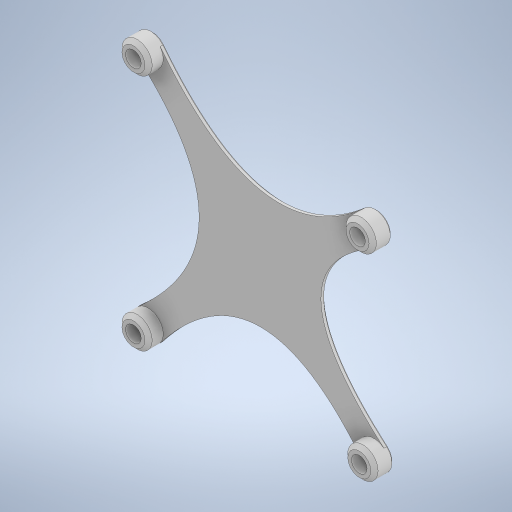
# Autodesk Inventor part: TinyFan_Extrusion_Top
Saved by Autodesk Inventor 2023.1 (Build 271208000, 208)
## iProperties
Created: 2022-09-15
Part Number: TinyFan_Extrusion_Top
Material: Generisch
Document SubType Name: Modeling
Designer: Rama
Density: 1 g/cm^3
Appearance: Vorgabe
Author: Rama
Autodesk Inventor part; units mm, degrees
ref_plane "YZ Plane" through (0, 0, 0) normal (1, 0, 0) x (0, 1, 0)
ref_plane "XZ Plane" through (0, 0, 0) normal (0, 1, 0) x (-1, 0, 0)
ref_plane "XY Plane" through (0, 0, 0) normal (0, 0, 1) x (1, 0, 0)
sketch "Skizze1" plane through (0, 0, 0) normal (0, 0, 1) x (1, 0, 0)
  circle A0 centre (-25.837, 27.4295) radius 1.65 projected
  line L0 (-38.2086, 5.3216) -> (-37.4869, 5.3204) projected
  line L1 (-37.4869, 5.3204) -> (-37.4918, 2.4829) projected
  line L2 (-37.4918, 2.4829) -> (-35.7716, 2.4799) projected
  line L3 (-35.7716, 2.4799) -> (-35.7668, 5.1987) projected
  line L4 (-35.7668, 5.1987) -> (-35.0451, 5.1975) projected
  line L5 (-35.0451, 5.1975) -> (-35.0499, 2.4787) projected
  line L6 (-35.0499, 2.4787) -> (-32.1136, 2.4735) projected
  line L7 (-32.1136, 2.4735) -> (-32.115, 1.6628) projected
  line L8 (-32.115, 1.6628) -> (-38.215, 1.6735) projected
  line L9 (-38.215, 1.6735) -> (-38.2086, 5.3216) projected
  line L10 (-35.0952, -3.6509) -> (-32.1243, -3.6561) projected
  line L11 (-32.1243, -3.6561) -> (-32.1256, -4.4273) projected
  line L12 (-32.1256, -4.4273) -> (-34.7356, -4.4227) projected
  spline S0 degree 2 poles (-34.7356, -4.4227) (-35.052, -4.4222) (-35.5959, -4.4805) (-35.7592, -4.5692) knots 0 0 0 1 2 2 2 projected
  spline S1 degree 2 poles (-35.7592, -4.5692) (-35.9323, -4.6628) (-36.101, -4.9987) (-36.1015, -5.2854) knots 0 0 0 1 2 2 2 projected
  spline S2 degree 2 poles (-36.1015, -5.2854) (-36.102, -5.5721) (-35.7966, -6.1807) (-35.5499, -6.4728) knots 0 0 0 1 2 2 2 projected
  line L13 (-35.5499, -6.4728) -> (-32.1292, -6.4787) projected
  line L14 (-32.1292, -6.4787) -> (-32.1305, -7.2499) projected
  line L15 (-32.1305, -7.2499) -> (-36.708, -7.2419) projected
  line L16 (-36.708, -7.2419) -> (-36.7066, -6.4707) projected
  line L17 (-36.7066, -6.4707) -> (-36.1975, -6.4716) projected
  spline S3 degree 2 poles (-36.1975, -6.4716) (-36.5083, -6.125) (-36.8334, -5.4571) (-36.8327, -5.0815) knots 0 0 0 1 2 2 2 projected
  spline S4 degree 2 poles (-36.8327, -5.0815) (-36.8316, -4.4092) (-35.9405, -3.6495) (-35.0952, -3.6509) knots 0 0 0 1 2 2 2 projected
  line L18 (-36.71, -8.3739) -> (-32.1325, -8.3819) projected
  line L19 (-32.1325, -8.3819) -> (-32.1338, -9.153) projected
  line L20 (-32.1338, -9.153) -> (-36.7113, -9.145) projected
  line L21 (-36.7113, -9.145) -> (-36.71, -8.3739) projected
  line L22 (-32.1384, -11.773) -> (-32.1398, -12.5837) projected
  line L23 (-32.1398, -12.5837) -> (-37.5181, -12.5743) projected
  line L24 (-37.5181, -12.5743) -> (-37.5217, -14.6208) projected
  line L25 (-37.5217, -14.6208) -> (-38.2434, -14.6195) projected
  line L26 (-38.2434, -14.6195) -> (-38.2348, -9.7158) projected
  line L27 (-38.2348, -9.7158) -> (-37.5131, -9.7171) projected
  line L28 (-37.5131, -9.7171) -> (-37.5167, -11.7636) projected
  line L29 (-37.5167, -11.7636) -> (-32.1384, -11.773) projected
  line L30 (-38.2719, -8.3168) -> (-37.4711, -8.3182) projected
  line L31 (-37.4711, -8.3182) -> (-37.4727, -9.1931) projected
  line L32 (-37.4727, -9.1931) -> (-38.2735, -9.1917) projected
  line L33 (-38.2735, -9.1917) -> (-38.2719, -8.3168) projected
  line L34 (-36.695, 0.2274) -> (-36.6936, 1.0282) projected
  line L35 (-36.6936, 1.0282) -> (-30.4347, -1.4445) projected
  line L36 (-30.4347, -1.4445) -> (-30.4362, -2.27) projected
  line L37 (-30.4362, -2.27) -> (-32.3428, -1.4461) projected
  line L38 (-32.3428, -1.4461) -> (-36.7008, -3.0994) projected
  line L39 (-36.7008, -3.0994) -> (-36.6993, -2.269) projected
  line L40 (-36.6993, -2.269) -> (-33.306, -1.0242) projected
  line L41 (-33.306, -1.0242) -> (-36.695, 0.2274) projected
  line L42 (-32.103, 8.529) -> (-32.5874, 8.5299) projected
  spline S5 degree 2 poles (-32.5874, 8.5299) (-32.5184, 8.4358) (-32.2718, 8.119) (-32.1979, 7.9706) knots 0 0 0 1 2 2 2 projected
  spline S6 degree 2 poles (-32.1979, 7.9706) (-32.0895, 7.7677) (-31.9765, 7.3869) (-31.9771, 7.0409) knots 0 0 0 1 2 2 2 projected
  spline S7 degree 2 poles (-31.9771, 7.0409) (-31.9775, 6.7591) (-32.191, 6.2503) (-32.3841, 6.0579) knots 0 0 0 1 2 2 2 projected
  spline S8 degree 2 poles (-32.3841, 6.0579) (-32.5723, 5.8753) (-33.1263, 5.6538) (-33.4328, 5.6544) knots 0 0 0 1 2 2 2 projected
  spline S9 degree 2 poles (-33.4328, 5.6544) (-33.9074, 5.6552) (-34.5789, 6.0568) (-34.771, 6.4921) knots 0 0 0 1 2 2 2 projected
  spline S10 degree 2 poles (-34.771, 6.4921) (-34.9483, 6.878) (-35.0799, 7.9262) (-35.1134, 8.5343) knots 0 0 0 1 2 2 2 projected
  line L43 (-35.1134, 8.5343) -> (-35.2617, 8.5345) projected
  spline S11 degree 2 poles (-35.2617, 8.5345) (-35.5287, 8.535) (-35.8602, 8.3725) (-35.9543, 8.2243) knots 0 0 0 1 2 2 2 projected
  spline S12 degree 2 poles (-35.9543, 8.2243) (-36.0485, 8.0762) (-36.1086, 7.6512) (-36.109, 7.4238) knots 0 0 0 1 2 2 2 projected
  spline S13 degree 2 poles (-36.109, 7.4238) (-36.1094, 7.1569) (-35.9525, 6.4349) (-35.7999, 6.0737) knots 0 0 0 1 2 2 2 projected
  line L44 (-35.7999, 6.0737) -> (-35.8, 6.0292) projected
  line L45 (-35.8, 6.0292) -> (-36.586, 6.0306) projected
  spline S14 degree 2 poles (-36.586, 6.0306) (-36.6449, 6.2433) (-36.7918, 7.0394) (-36.7911, 7.4299) knots 0 0 0 1 2 2 2 projected
  spline S15 degree 2 poles (-36.7911, 7.4299) (-36.7903, 7.9045) (-36.6409, 8.5518) (-36.4476, 8.8085) knots 0 0 0 1 2 2 2 projected
  spline S16 degree 2 poles (-36.4476, 8.8085) (-36.2594, 9.0603) (-35.6608, 9.3064) (-35.2307, 9.3056) knots 0 0 0 1 2 2 2 projected
  line L46 (-35.2307, 9.3056) -> (-32.1016, 9.3002) projected
  line L47 (-32.1016, 9.3002) -> (-32.103, 8.529) projected
  line L48 (-35.0644, 13.9817) -> (-32.0935, 13.9765) projected
  line L49 (-32.0935, 13.9765) -> (-32.0948, 13.2054) projected
  line L50 (-32.0948, 13.2054) -> (-34.7049, 13.2099) projected
  spline S17 degree 2 poles (-34.7049, 13.2099) (-35.0212, 13.2105) (-35.5651, 13.1521) (-35.7284, 13.0634) knots 0 0 0 1 2 2 2 projected
  spline S18 degree 2 poles (-35.7284, 13.0634) (-35.9016, 12.9698) (-36.0702, 12.6339) (-36.0707, 12.3472) knots 0 0 0 1 2 2 2 projected
  spline S19 degree 2 poles (-36.0707, 12.3472) (-36.0712, 12.0605) (-35.7658, 11.452) (-35.5191, 11.1599) knots 0 0 0 1 2 2 2 projected
  line L51 (-35.5191, 11.1599) -> (-32.0984, 11.1539) projected
  line L52 (-32.0984, 11.1539) -> (-32.0998, 10.3828) projected
  line L53 (-32.0998, 10.3828) -> (-36.6772, 10.3907) projected
  line L54 (-36.6772, 10.3907) -> (-36.6759, 11.1619) projected
  line L55 (-36.6759, 11.1619) -> (-36.1667, 11.161) projected
  spline S20 degree 2 poles (-36.1667, 11.161) (-36.4775, 11.5076) (-36.8026, 12.1755) (-36.802, 12.5512) knots 0 0 0 1 2 2 2 projected
  spline S21 degree 2 poles (-36.802, 12.5512) (-36.8008, 13.2235) (-35.9097, 13.9832) (-35.0644, 13.9817) knots 0 0 0 1 2 2 2 projected
  circle A1 centre (-25.837, -24.3815) radius 1.65 projected
  circle A2 centre (22.931, 18.2855) radius 1.65 projected
  circle A3 centre (23.297, -24.3815) radius 1.65 projected
  arc A4 (-37.7973, 28.9208) -> (-39.6082, 27.5864) centre (-37.7217, 26.9222) ccw projected
  arc A5 (-39.6082, 27.5864) -> (-39.8919, 25.917) centre (-34.8919, 25.926) ccw projected
  line L56 (-39.8919, 25.917) -> (-39.8874, 23.4424) projected
  line L57 (-39.8874, 23.4424) -> (-39.478, 23.4424) projected
  arc A6 (-39.478, 21.4424) -> (-39.478, 23.4424) centre (-34.8856, 22.4424) ccw projected
  line L58 (-39.478, 21.4424) -> (-39.8838, 21.4424) projected
  line L59 (-39.8838, 21.4424) -> (-39.8061, -21.5576) projected
  line L60 (-39.8061, -21.5576) -> (-39.3966, -21.5576) projected
  arc A7 (-39.3966, -23.5576) -> (-39.3966, -21.5576) centre (-34.8043, -22.5576) ccw projected
  line L61 (-39.3966, -23.5576) -> (-39.8025, -23.5576) projected
  line L62 (-39.8025, -23.5576) -> (-39.798, -26.0503) projected
  arc A8 (-39.798, -26.0503) -> (-39.5082, -27.7186) centre (-34.798, -26.0413) ccw projected
  arc A9 (-39.5082, -27.7186) -> (-37.6925, -29.0465) centre (-37.6241, -27.0477) ccw projected
  line L63 (-37.6925, -29.0465) -> (-31.8925, -29.036) projected
  spline S22 degree 2 poles (-31.8925, -29.036) (-30.8606, -29.0341) (-25.3454, -28.3512) knots -2 -2 -2 -1 -1 -1 projected
  arc A10 (-25.3454, -28.3512) -> (-22.6346, -26.7782) centre (-25.837, -24.3815) ccw projected
  spline S23 degree 2 poles (-22.6346, -26.7782) (-1.453, 1.524) (20.1144, -26.8045) knots -2 -2 -2 -1 -1 -1 projected
  arc A11 (20.1144, -26.8045) -> (25.8626, -21.3127) centre (23.297, -24.3815) ccw projected
  arc A12 (24.7305, 14.7131) -> (20.2403, 21.2453) centre (22.931, 18.2855) ccw projected
  spline S24 degree 2 poles (20.2403, 21.2453) (-1.453, 1.524) (-22.6346, 29.8262) knots -2 -2 -2 -1 -1 -1 projected
  arc A13 (-22.6346, 29.8262) -> (-27.9876, 30.8022) centre (-25.837, 27.4295) ccw projected
  spline S25 degree 2 poles (-27.9876, 30.8022) (-30.9185, 28.9332) (-31.9973, 28.9313) knots -2 -2 -2 -1 -1 -1 projected
  line L64 (-31.9973, 28.9313) -> (-37.7973, 28.9208) projected
  circle A14 centre (-25.837, 27.4295) radius 1.7
  circle A15 centre (-25.837, -24.3815) radius 1.7
  circle A16 centre (23.297, -24.3815) radius 1.7
  circle A17 centre (22.931, 18.2855) radius 1.7
  circle A18 centre (-25.837, 27.4295) radius 3.3
  circle A19 centre (22.931, 18.2855) radius 3.3
  circle A20 centre (23.297, -24.3815) radius 3.3
  circle A21 centre (-25.837, -24.3815) radius 3.3
  line L65 (-28.0198, -21.9065) -> (-1.453, 1.524) construction
  line L66 (-1.453, 1.524) -> (-28.0198, 24.9545) construction
  spline S26 degree 2 poles (-28.0198, -21.9065) (-1.453, 1.524) (-28.0198, 24.9545) knots 1 1 1 2 2 2
  line L67 (-23.2346, 29.4587) -> (-1.453, 1.524) construction
  line L68 (-1.453, 1.524) -> (20.77, 20.7795) construction
  spline S27 degree 2 poles (-23.2346, 29.4587) (-1.453, 1.524) (20.77, 20.7795) knots 1 1 1 2 2 2
  line L69 (-23.2346, -26.4107) -> (-1.453, 1.524) construction
  line L70 (-1.453, 1.524) -> (20.7111, -26.4317) construction
  spline S28 degree 2 poles (-23.2346, -26.4107) (-1.453, 1.524) (20.7111, -26.4317) knots 1 1 1 2 2 2
  line L71 (25.4629, -21.8918) -> (-1.453, 1.524) construction
  line L72 (-1.453, 1.524) -> (24.4854, 15.3745) construction
  spline S29 degree 2 poles (25.4629, -21.8918) (-1.453, 1.524) (24.4854, 15.3745) knots 1 1 1 2 2 2
  spline S30 degree 2 poles (25.8626, -21.3127) (21.9132, -18.0109) (19.0822, -14.9107) knots -2 -2 -2 -1.855416 -1.855416 -1.855416 projected
  spline S31 degree 2 poles (17.22, 9.815) (18.4126, 10.8679) (19.8732, 11.8725) knots 1.825455 1.825455 1.825455 1.896249 1.896249 1.896249 projected
  spline S32 degree 2 poles (17.22, -12.7436) (6.6116, 0.4487) (17.22, 9.815) knots -1.804293 -1.804293 -1.804293 -1.174545 -1.174545 -1.174545 projected
  spline S33 degree 2 poles (19.8732, 11.8725) (22.0139, 13.3447) (24.7305, 14.7131) knots -1.103751 -1.103751 -1.103751 -1 -1 -1 projected
  spline S34 degree 2 poles (19.0822, -14.9107) (18.0812, -13.8146) (17.22, -12.7436) knots 1.144584 1.144584 1.144584 1.195707 1.195707 1.195707 projected
  point P0 (0, 0)
  point P1 (24.4854, 15.3745)
  point P2 (20.77, 20.7795)
  dimension "d5" = 6.6
  dimension "d0" = 3.4
  dimension "d1" = 3.4
  dimension "d2" = 3.4
  dimension "d3" = 3.4
  dimension "d4" = 1.6
  dimension "d6" = 6.6
  dimension "d7" = 6.6
  dimension "d8" = 6.6
  dimension "d9" = 51.811
  dimension "d10" = 25.9055
  dimension "d11" = 48.768
  dimension "d12" = 24.384
  constraints: 11 coincident, 7 centre point, 21 other
  measures "d0" diameter of A14
  measures "d1" diameter of A15
  measures "d2" diameter of A16
  measures "d3" diameter of A17
  measures "d6" diameter of A19
  measures "d7" diameter of A20
  measures "d8" diameter of A21
  measures "d9" distance of A1.centre A0.centre
  measures "d10" vertical distance of L71.end A1.centre
  measures "d11" horizontal distance of A2.centre A0.centre
  measures "d12" horizontal distance of L67.end A0.centre
extrude "Extrusion1" add sketch "Skizze1" along normal blind 1 contours A18 | A18 S27 A19 S29 A20 S28 A21 S26 | A19 | A21 | A20
sketch "Skizze2" plane through (0, 0, 1) normal (0, 0, 1) x (1, 0, 0)
  circle A0 centre (-25.837, 27.4295) radius 1.7 projected
  circle A1 centre (22.931, 18.2855) radius 1.7 projected
  circle A2 centre (23.297, -24.3815) radius 1.7 projected
  circle A3 centre (-25.837, -24.3815) radius 1.7 projected
  circle A4 centre (-25.837, 27.4295) radius 1.7 projected
  circle A5 centre (-25.837, 27.4295) radius 3.3
  circle A6 centre (22.931, 18.2855) radius 3.3
  circle A7 centre (23.297, -24.3815) radius 3.3
  circle A8 centre (-25.837, -24.3815) radius 3.3
  point P0 (0, 0)
  dimension "d15" = 6.6
  dimension "d16" = 6.6
  dimension "d17" = 6.6
  dimension "d18" = 6.6
  constraints: 4 centre point, 4 coincident
  measures "d15" diameter of A5
  measures "d16" diameter of A6
  measures "d17" diameter of A7
  measures "d18" diameter of A8
extrude "Extrusion2" add sketch "Skizze2" along normal blind 3.2
chamfer "Fase1" distance 0.4 angle 45 12 edges at (-1.3426, 13.3215, 0) (-28.0988, 29.8325, 0) (-14.7364, 1.524, 0) (-28.0988, -26.7845, 0) (-1.3574, -12.4486, 0) (25.5766, -26.7676, 0) (11.7606, -0.8673, 0) (25.6505, 20.1549, 0) (-27.537, 27.4295, 0) (-27.537, -24.3815, 0) (21.597, -24.3815, 0) (21.231, 18.2855, 0)
chamfer "Fase2" distance 0.8 angle 45 4 edges at (-29.137, 27.4295, 4.2) (19.631, 18.2855, 4.2) (19.997, -24.3815, 4.2) (-29.137, -24.3815, 4.2)
equation "\"d6\" = d5"
equation "\"d7\" = d5"
equation "\"d8\" = d5"
equation "\"d10\" = 0.5 * d9"
equation "\"d12\" = 0.5 * d11"
